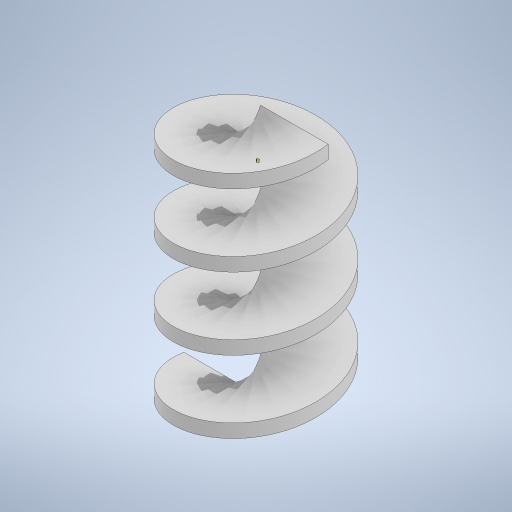
# Autodesk Inventor part: bobina
Saved by Autodesk Inventor 2023 (Build 270158000, 158)
## iProperties
Created: 2022-04-04
Part Number: bobina
Material: Genérico
Document SubType Name: Modeling
Designer: isaac
Density: 1 g/cm^3
Appearance: Valor por defecto
Author: isaac
Autodesk Inventor part; units mm, degrees
ref_plane "YZ Plane" through (0, 0, 0) normal (1, 0, 0) x (0, 1, 0)
ref_plane "XZ Plane" through (0, 0, 0) normal (0, 1, 0) x (-1, 0, 0)
ref_plane "XY Plane" through (0, 0, 0) normal (0, 0, 1) x (1, 0, 0)
sketch "Boceto3" plane through (0, 0, 0) normal (0, 0, 1) x (1, 0, 0)
  line L0 (1, 1.5) -> (16, 1.5)
  line L1 (16, 1.5) -> (16, -1.5)
  line L2 (16, -1.5) -> (1, -1.5)
  line L3 (1, -1.5) -> (1, 1.5)
  point P0 (0, 0)
  point P1 (1, 0)
  dimension "d4" = 3
  dimension "d5" = 15
  dimension "d6" = 16
  constraints: 8 end point, 2 parallel, 1 horizontal, 1 horizontal alignment, 1 midpoint, 1 perpendicular
  measures "d4" distance between parallel lines of L2 L0
  measures "d5" distance between parallel lines of L1 L3
  measures "d6" distance from line of point (0, 0) L1
coil "Bobina1" sketch "Boceto3" operation add axis through (0, -10, 0) along (0, -1, 0) pitch 16 turns 3.5 hand right
